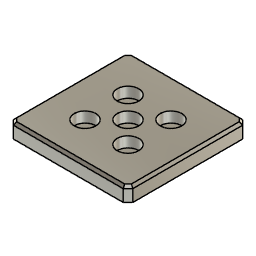
Magnetic Base (Autodesk Fusion 360 design; units mm, degrees)
Autodesk Fusion 360 part; units mm, degrees
sketch "Sketch1" plane through (0, 0, 0) normal (0, 0, 1) x (1, 0, 0)
  line L0 (-100, 100) -> (0, 100)
  line L1 (0, 100) -> (0, 0)
  line L2 (0, 0) -> (-100, 0)
  line L3 (-100, 0) -> (-100, 100)
  constraint horizontal L0
  constraint vertical L1
  constraint horizontal L2
  constraint vertical L3
  constraint coincident L1.end L2.start
extrude "Extrude1" add sketch "Sketch1" along normal blind 3 makes body 1
sketch "Sketch2" plane through (0, 0, 3) normal (0, 0, 1) x (-1, 0, 0)
  line L0 (100, 0) -> (0, 0)
  line L1 (0, 0) -> (0, -100)
  line L2 (0, -100) -> (100, -100)
  line L3 (100, -100) -> (100, 0)
  circle A0 centre (50, -50) radius 2.75
  dimension "d3" = 5.5
  measures "d3" diameter of A0
extrude "Extrude2" add sketch "Sketch2" along normal blind 1 contours L0 L1 L2 L3 | A0 bodies 1
sketch "Sketch3" plane through (0, 0, 4) normal (0, 0, 1) x (-1, 0, 0)
  line L0 (100, -100) -> (100, 0)
  line L1 (100, 0) -> (0, 0)
  line L2 (0, 0) -> (0, -100)
  line L3 (0, -100) -> (100, -100)
  circle A0 centre (50, -50) radius 2.75
  dimension "d6" = 5.5
  measures "d6" diameter of A0
extrude "Extrude3" cut sketch "Sketch3" against normal blind 3.25 contours A0 bodies 1
chamfer "Chamfer1" distance 0.5 angle 45 1 edges at (-47.4361, 49.0056, 4) on bodies 1
sketch "Sketch4" plane through (0, 0, 0) normal (0, 0, 1) x (1, 0, 0)
  line L0 (0, 0) -> (-25, 0)
  line L1 (-25, 0) -> (-25, 25)
  line L2 (-25, 25) -> (0, 25)
  line L3 (0, 25) -> (0, 0)
  constraint horizontal L0
  constraint vertical L1
  constraint horizontal L2
  constraint vertical L3
  constraint coincident L0.start L3.end
extrude "Extrude4" add sketch "Sketch4" along normal blind 3 separate body makes body 2
extrude "Extrude5" add 1 faces at (-8.3333, 8.3333, 3) along direction (0, 0, 1) blind 1 on bodies 2 bodies 2
sketch "Sketch5" plane through (0, 0, 4) normal (0, 0, 1) x (-1, 0, 0)
  line L0 (0, -25) -> (25, -25)
  line L1 (25, -25) -> (25, 0)
  line L2 (25, 0) -> (0, 0)
  line L3 (0, 0) -> (0, -25)
  circle A0 centre (12.5, -12.5) radius 2.75
  dimension "d14" = 5.5
  measures "d14" diameter of A0
extrude "Extrude6" cut sketch "Sketch5" against normal blind 3.25 contours A0 bodies 2
chamfer "Chamfer2" distance 0.5 angle 45 1 edges at (-9.9361, 11.5056, 4) on bodies 2
chamfer "Chamfer3" distance 0.5 angle 45 4 edges at (-12.5, 0, 4) (-25, 12.5, 4) (0, 12.5, 4) (-12.5, 25, 4) on bodies 2
sketch "Sketch6" plane through (0, 0, 4) normal (0, 0, 1) x (-1, 0, 0)
  circle A0 centre (12.5, -12.5) radius 3.25
  line L0 (0.5, -24.5) -> (24.5, -24.5)
  line L1 (24.5, -24.5) -> (24.5, -0.5)
  line L2 (24.5, -0.5) -> (0.5, -0.5)
  line L3 (0.5, -0.5) -> (0.5, -24.5)
  circle A1 centre (5, -5) radius 2.75
  circle A2 centre (20, -5) radius 2.75
  circle A3 centre (5, -20) radius 2.75
  circle A4 centre (20, -20) radius 2.75
  dimension "d19" = 5.5
  dimension "d20" = 5.5
  dimension "d21" = 5.5
  dimension "d22" = 5.5
  measures "d19" diameter of A1
  measures "d20" diameter of A2
  measures "d21" diameter of A3
  measures "d22" diameter of A4
extrude "Extrude7" cut sketch "Sketch6" against normal blind 3.25 contours A1 | A2 | A3 | A4 bodies 2
chamfer "Chamfer4" distance 0.5 angle 45 4 edges at (-2.4361, 4.0056, 4) (-17.4361, 4.0056, 4) (-17.4361, 19.0056, 4) (-2.4361, 19.0056, 4) on bodies 2
sketch "Sketch7" plane through (0, 0, 0) normal (0, 0, 1) x (1, 0, 0)
  line L0 (-25, 25) -> (0, 25)
  line L1 (0, 25) -> (0, 0)
  line L2 (0, 0) -> (-25, 0)
  line L3 (-25, 0) -> (-25, 25)
  constraint horizontal L0
  constraint vertical L1
  constraint horizontal L2
  constraint vertical L3
  constraint coincident L1.end L2.start
extrude "Extrude8" add sketch "Sketch7" along normal blind 3 separate body makes body 3
chamfer "Chamfer5" distance 1 angle 45 4 edges at (0, 25, 1.5) (0, 0, 1.5) (-25, 0, 1.5) (-25, 25, 1.5) on bodies 3
chamfer "Chamfer6" distance 0.5 angle 45 8 edges at (-0.5, 0.5, 3) (-12.5, 0, 3) (-24.5, 0.5, 3) (-25, 12.5, 3) (0, 12.5, 3) (-0.5, 24.5, 3) (-12.5, 25, 3) (-24.5, 24.5, 3) on bodies 3
sketch "Sketch8" plane through (0, 0, 3) normal (0, 0, 1) x (-1, 0, 0)
  line L0 (1.2071, -24.5) -> (23.7929, -24.5)
  line L1 (23.7929, -24.5) -> (24.5, -23.7929)
  line L2 (24.5, -23.7929) -> (24.5, -1.2071)
  line L3 (24.5, -1.2071) -> (23.7929, -0.5)
  line L4 (23.7929, -0.5) -> (1.2071, -0.5)
  line L5 (1.2071, -0.5) -> (0.5, -1.2071)
  line L6 (0.5, -1.2071) -> (0.5, -23.7929)
  line L7 (0.5, -23.7929) -> (1.2071, -24.5)
  circle A0 centre (12.5, -12.5) radius 2.25
  circle A1 centre (17, -17) radius 2.25
  circle A2 centre (8, -17) radius 2.25
  circle A3 centre (17, -8) radius 2.25
  circle A4 centre (8, -8) radius 2.25
  dimension "d30" = 4.5
  dimension "d31" = 4.5
  dimension "d32" = 4.5
  dimension "d33" = 4.5
  dimension "d34" = 4.5
  measures "d30" diameter of A0
  measures "d31" diameter of A1
  measures "d32" diameter of A2
  measures "d33" diameter of A3
  measures "d34" diameter of A4
extrude "Extrude9" cut sketch "Sketch8" against normal blind 2.2 contours A0 | A1 | A2 | A3 | A4 bodies 3
hidden bodies 1 2
